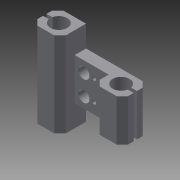
# Autodesk Inventor part: ChimeraXCarriage2
Saved by Autodesk Inventor 2015 (Build 190159000, 159)
## iProperties
Created: 2014-12-05
Part Number: ChimeraXCarriage2
Material: Generic
Document SubType Name: Modeling
Designer: Jack
Density: 1 g/cm^3
Appearance: Default
Author: Jack
Autodesk Inventor part; units mm, degrees
ref_plane "YZ Plane" through (0, 0, 0) normal (1, 0, 0) x (0, 1, 0)
ref_plane "XZ Plane" through (0, 0, 0) normal (0, 1, 0) x (-1, 0, 0)
ref_plane "XY Plane" through (0, 0, 0) normal (0, 0, 1) x (1, 0, 0)
sketch "Sketch1" plane through (0, 0, 0) normal (0, 0, 1) x (1, 0, 0)
  arc A0 (-7.3485, -1.5) -> (-7.3485, 1.5) centre (0, 0) ccw
  arc A1 (62.3485, 1.5) -> (62.3485, -1.5) centre (55, 0) ccw
  line L0 (-12.5, 11.5) -> (67.5, 11.5)
  line L1 (67.5, -11.5) -> (-12.5, -11.5)
  line L2 (-12.5, 1.5) -> (-7.3485, 1.5)
  line L3 (-12.5, -1.5) -> (-7.3485, -1.5)
  line L4 (-12.5, -11.5) -> (-12.5, -1.5)
  line L5 (-12.5, 1.5) -> (-12.5, 11.5)
  line L6 (67.5, 1.5) -> (62.3485, 1.5)
  line L7 (67.5, -1.5) -> (62.3485, -1.5)
  line L8 (67.5, 11.5) -> (67.5, 1.5)
  line L9 (67.5, -1.5) -> (67.5, -11.5)
  dimension "d0" = 15
  dimension "d1" = 15
  dimension "d2" = 55
  dimension "d3" = 11.5
  dimension "d4" = 11.5
  dimension "d7" = 1.5
  dimension "d8" = 3
  dimension "d9" = 12.5
  dimension "d10" = 12.5
  constraints: 20 end point, 6 perpendicular, 4 point on circle, 3 horizontal, 3 horizontal alignment, 2 centre point, 2 vertical, 2 vertical alignment, 1 coincident, 1 parallel
  measures "d0" diameter of A0
  measures "d1" diameter of A1
  measures "d2" distance of point (0, 0) A1.centre
  measures "d3" distance from line of point (0, 0) L1
  measures "d4" distance from line of L0 point (0, 0)
  measures "d7" distance from line of A1.centre L7
  measures "d8" distance between parallel lines of L6 L7
  measures "d9" distance from line of point (0, 0) L5
  measures "d10" distance from line of L8 A1.centre
extrude "Extrusion1" add sketch "Sketch1" along normal blind 75
chamfer "Chamfer1" distance 5 angle 45 4 edges at (-12.5, 11.5, 37.5) (-12.5, -11.5, 37.5) (67.5, 11.5, 37.5) (67.5, -11.5, 37.5)
sketch "Sketch2" plane through (0, 0, 75) normal (0, 0, 1) x (1, 0, 0)
  arc A0 (62.3485, 1.5) -> (62.3485, -1.5) centre (55, 0) ccw projected
  line L0 (62.5, 11.5) -> (-7.5, 11.5) projected
  arc A1 (-7.3485, -1.5) -> (-7.3485, 1.5) centre (0, 0) ccw projected
  line L1 (-7.5, -11.5) -> (62.5, -11.5) projected
  line L2 (-7.5, -11.5) -> (62.5, -11.5) projected
  line L3 (7.5, -11.5) -> (12.5, -6.5)
  line L4 (12.5, -6.5) -> (12.5, 1.5)
  line L5 (12.5, 1.5) -> (42.5, 1.5)
  line L6 (42.5, 1.5) -> (42.5, -6.5)
  line L7 (42.5, -6.5) -> (47.5, -11.5)
  dimension "d16" = 135
  dimension "d17" = 12.5
  dimension "d18" = 12.5
  dimension "d19" = 5
  dimension "d20" = 10
  constraints: 10 end point, 4 perpendicular, 2 point on line, 1 horizontal alignment
  measures "d16" angle of L1 L7
  measures "d17" distance from line of L4 A1.centre
  measures "d18" distance from line of A0.centre L6
  measures "d19" horizontal distance of L3.start L3.end
  measures "d20" distance between parallel lines of L0 L5
extrude "Extrusion2" cut sketch "Sketch2" against normal up to next
sketch "Sketch3" plane through (12.5, 1.5, 75) normal (0, -1, 0) x (1, 0, 0)
  line L0 (30, -75) -> (0, -75) projected
  line L1 (0, 0) -> (0, -75) projected
  circle A0 centre (17, -46.5) radius 1.75
  circle A1 centre (17, -28.5) radius 1.75
  point P0 (-12.5, -75)
  dimension "d23" = 18
  dimension "d24" = 17
  dimension "d25" = 28.5
  dimension "d26" = 3.5
  constraints: 2 centre point, 1 equal radius, 1 vertical alignment
  measures "d23" distance of A1.centre A0.centre
  measures "d24" distance from line of L1 A1.centre
  measures "d25" distance from line of L0 A0.centre
  measures "d26" diameter of A0
extrude "Extrusion3" cut sketch "Sketch3" against normal up to next
sketch "Sketch4" plane through (12.5, 1.5, 75) normal (0, -1, 0) x (1, 0, 0)
  circle A0 centre (17, -46.5) radius 1.75 projected
  circle A1 centre (17, -28.5) radius 1.75 projected
  circle A2 centre (8, -46.5) radius 5
  circle A3 centre (8, -28.5) radius 5
  point P0 (-12.5, -75)
  dimension "d29" = 10
  dimension "d30" = 9
  constraints: 2 centre point, 2 horizontal alignment, 1 equal radius, 1 vertical alignment
  measures "d29" diameter of A2
  measures "d30" distance of A0.centre A2.centre
extrude "Extrusion4" cut sketch "Sketch4" against normal up to next contours A2 | A3
sketch "Sketch5" plane through (0, 0, 75) normal (0, 0, 1) x (1, 0, 0)
  line L0 (12.5, 1.5) -> (42.5, 1.5) projected
  line L1 (42.5, 1.5) -> (42.5, -6.5) projected
  line L2 (42.5, -6.5) -> (47.5, -11.5) projected
  line L3 (47.5, -11.5) -> (62.5, -11.5) projected
  line L4 (67.5, -6.5) -> (62.5, -11.5) projected
  line L5 (67.5, -6.5) -> (67.5, -1.5) projected
  line L6 (67.5, -1.5) -> (62.3485, -1.5) projected
  arc A0 (62.3485, 1.5) -> (62.3485, -1.5) centre (55, 0) ccw projected
  line L7 (62.3485, 1.5) -> (67.5, 1.5) projected
  line L8 (67.5, 1.5) -> (67.5, 6.5) projected
  line L9 (62.5, 11.5) -> (67.5, 6.5) projected
  line L10 (62.5, 11.5) -> (-7.5, 11.5) projected
  line L11 (12.5, 1.5) -> (12.5, 11.5)
  constraints: 2 end point, 1 perpendicular, 1 point on line
extrude "Extrusion5" cut sketch "Sketch5" against normal blind 19
sketch "Sketch6" plane through (0, 0, 0) normal (0, 0, -1) x (-1, 0, 0)
  line L0 (-62.5, 11.5) -> (7.5, 11.5) projected
  line L1 (-67.5, 6.5) -> (-62.5, 11.5) projected
  line L2 (-67.5, 1.5) -> (-67.5, 6.5) projected
  line L3 (-62.3485, 1.5) -> (-67.5, 1.5) projected
  arc A0 (-62.3485, -1.5) -> (-62.3485, 1.5) centre (-55, 0) ccw projected
  line L4 (-67.5, -1.5) -> (-62.3485, -1.5) projected
  line L5 (-67.5, -6.5) -> (-67.5, -1.5) projected
  line L6 (-62.5, -11.5) -> (-67.5, -6.5) projected
  line L7 (-47.5, -11.5) -> (-62.5, -11.5) projected
  line L8 (-47.5, -11.5) -> (-42.5, -6.5) projected
  line L9 (-42.5, -6.5) -> (-42.5, 1.5) projected
  line L10 (-42.5, 1.5) -> (-12.5, 1.5) projected
  line L11 (-12.5, 1.5) -> (-12.5, 11.5)
  constraints: 2 end point, 1 perpendicular, 1 point on line
extrude "Extrusion6" cut sketch "Sketch6" against normal blind 19
body "Solid1"
